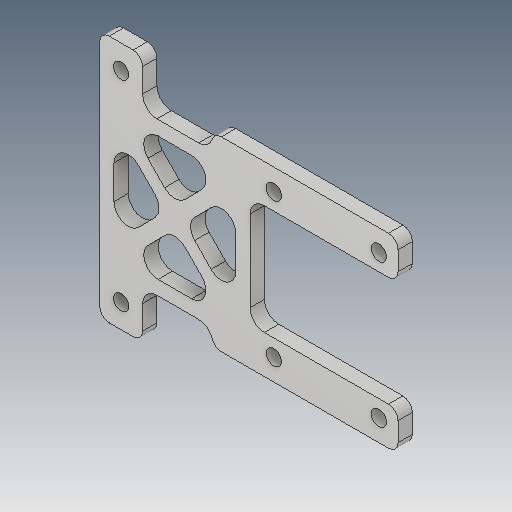
# Autodesk Inventor part: 肩ピッチ固定板_アルミ(A2017)_t3
Saved by Autodesk Inventor 2019.4 (Build 234330000, 330)
## iProperties
Created: 2019-06-27
Part Number: 肩ピッチ固定板_アルミ(A2017)_t3
Material: アルミニウム 2014-T6
Document SubType Name: Modeling
Designer: 長谷川翔一
Density: 2.78927 g/cm^3
Appearance: サテン
Mass: 14.0844 g
Surface Area: 44.3653 cm^2
Volume: 5.04948 cm^3
Author: 長谷川翔一
Autodesk Inventor part; units mm, degrees
ref_plane "YZ Plane" through (0, 0, 0) normal (1, 0, 0) x (0, 1, 0)
ref_plane "XZ Plane" through (0, 0, 0) normal (0, 1, 0) x (-1, 0, 0)
ref_plane "XY Plane" through (0, 0, 0) normal (0, 0, 1) x (1, 0, 0)
sketch "スケッチ1" plane through (0, 0, 0) normal (0, 0, 1) x (1, 0, 0)
  line L0 (7.25, -16) -> (-7.25, -16)
  line L1 (-16.25, -16) -> (-16.25, 16)
  line L2 (-7.25, 16) -> (7.25, 16)
  line L3 (16.25, -16) -> (-16.25, 16) construction
  line L4 (-16.25, -16) -> (16.25, 16) construction
  line L5 (16.25, 0) -> (46.25, 0) construction
  line L6 (46.25, -10.5) -> (16.25, -10.5) construction
  line L7 (16.25, 10.5) -> (46.25, 10.5) construction
  line L8 (46.25, 10.5) -> (46.25, -10.5) construction
  line L9 (46.25, -10.5) -> (16.25, 10.5) construction
  line L10 (16.25, -10.5) -> (46.25, 10.5) construction
  line L11 (46.25, 11.5) -> (15.25, 11.5)
  line L12 (15.25, 11.5) -> (15.25, -11.5)
  line L13 (15.25, -11.5) -> (46.25, -11.5)
  line L14 (46.25, 19.5) -> (7.25, 19.5)
  line L15 (7.25, -19.5) -> (46.25, -19.5)
  line L16 (46.25, 11.5) -> (46.25, 19.5)
  line L17 (46.25, -11.5) -> (46.25, -19.5)
  line L18 (16.25, 10.5) -> (16.25, -10.5) construction
  line L19 (7.25, 19.5) -> (7.25, 16)
  line L20 (7.25, -16) -> (7.25, -19.5)
  line L21 (-16.25, -16) -> (-16.25, -26)
  line L22 (-16.25, -26) -> (-7.25, -26)
  line L23 (-7.25, 26) -> (-16.25, 26)
  line L24 (-16.25, 26) -> (-16.25, 16)
  line L25 (-11.75, 26) -> (-11.75, -26) construction
  line L26 (-11.75, 0) -> (-16.25, 0) construction
  circle A0 centre (-11.75, -21) radius 1.6
  line L27 (-7.25, -26) -> (-7.25, -16)
  line L28 (-7.25, 16) -> (-7.25, 26)
  circle A1 centre (-11.75, 21) radius 1.6
  line L29 (46.25, 10.5) -> (16.25, 10.5) construction
  line L30 (31.25, 10.5) -> (31.25, 19.5) construction
  line L31 (31.25, 15) -> (46.25, 15) construction
  circle A2 centre (37.05, 15) radius 1.6 construction
  circle A3 centre (42.25, 15) radius 1.6
  circle A4 centre (25.45, 15) radius 1.6 construction
  circle A5 centre (20.25, 15) radius 1.6
  circle A6 centre (37.05, -15) radius 1.6 construction
  circle A7 centre (42.25, -15) radius 1.6
  circle A8 centre (25.45, -15) radius 1.6 construction
  circle A9 centre (20.25, -15) radius 1.6
  point P0 (0, 0)
  point P1 (31.25, 0)
  dimension "d21" = 32.5
  dimension "d22" = 32
  dimension "d24" = 30
  dimension "d25" = 21
  dimension "d26" = 1
  dimension "d28" = 30
  dimension "d30" = 9
  dimension "d32" = 9
  dimension "d33" = 3.2
  dimension "d34" = 5
  dimension "d35" = 10
  dimension "d36" = 8
  dimension "d37" = 31
  dimension "d38" = 3.5
  dimension "d39" = 35.5
  dimension "d40" = 9
  dimension "d41" = 3.2
  dimension "d42" = 3.2
  dimension "d43" = 4
  dimension "d44" = 31
  dimension "d46" = 2
  constraints: 64 end point, 11 midpoint, 10 centre point, 9 perpendicular, 7 symmetric about line, 6 parallel, 6 point on line, 3 horizontal, 2 collinear, 2 vertical, 7 other
  measures "d21" distance of L1.end L4.end
  measures "d22" distance of L1.start L1.end
  measures "d24" distance of L7.start L7.end
  measures "d25" distance of L6.end L7.start
  measures "d26" distance between parallel lines of L7 L11
  measures "d28" distance between parallel lines of L8 L18
  measures "d30" distance of L21.end L22.end
  measures "d32" distance of L23.start L23.end
  measures "d33" diameter of A0
  measures "d34" distance from line of L22 A0.centre
  measures "d35" distance between parallel lines of L0 L22
  measures "d36" distance between parallel lines of L15 L13
  measures "d37" distance between parallel lines of L11 L15
  measures "d38" distance between parallel lines of L15 L0
  measures "d39" distance between parallel lines of L15 L2
  measures "d40" distance of L30.start L30.end
  measures "d41" diameter of A2
  measures "d42" diameter of A3
  measures "d43" distance from line of L16 A3.centre
  measures "d44" distance from line of L31.end L12
extrude "押し出し1" add sketch "スケッチ1" along normal blind 3
fillet "フィレット1" radius 2 10 edges at (7.25, 19.5, 1.5) (-7.25, 26, 1.5) (-16.25, 26, 1.5) (46.25, 19.5, 1.5) (46.25, 11.5, 1.5) (46.25, -11.5, 1.5) (46.25, -19.5, 1.5) (7.25, -19.5, 1.5) (-7.25, -26, 1.5) (-16.25, -26, 1.5)
fillet "フィレット2" radius 3 6 edges at (15.25, -11.5, 1.5) (15.25, 11.5, 1.5) (7.25, 16, 1.5) (7.25, -16, 1.5) (-7.25, -16, 1.5) (-7.25, 16, 1.5)
sketch "スケッチ2" plane through (0, 0, 3) normal (0, 0, 1) x (1, 0, 0)
  arc A0 (-16.25, -24) -> (-14.25, -26) centre (-14.25, -24) ccw projected
  line L0 (-14.25, -26) -> (-9.25, -26) projected
  arc A1 (-9.25, -26) -> (-7.25, -24) centre (-9.25, -24) ccw projected
  line L1 (-7.25, -24) -> (-7.25, -19) projected
  arc A2 (-4.25, -16) -> (-7.25, -19) centre (-4.25, -19) ccw projected
  line L2 (-4.25, -16) -> (4.4803, -16) projected
  arc A3 (7.3421, -18.1) -> (4.4803, -16) centre (4.4803, -19) ccw projected
  arc A4 (7.3421, -18.1) -> (9.25, -19.5) centre (9.25, -17.5) ccw projected
  line L3 (9.25, -19.5) -> (44.25, -19.5) projected
  arc A5 (44.25, -19.5) -> (46.25, -17.5) centre (44.25, -17.5) ccw projected
  line L4 (46.25, -17.5) -> (46.25, -13.5) projected
  arc A6 (46.25, -13.5) -> (44.25, -11.5) centre (44.25, -13.5) ccw projected
  line L5 (44.25, -11.5) -> (18.25, -11.5) projected
  arc A7 (15.25, -8.5) -> (18.25, -11.5) centre (18.25, -8.5) ccw projected
  line L6 (15.25, -8.5) -> (15.25, 8.5) projected
  arc A8 (18.25, 11.5) -> (15.25, 8.5) centre (18.25, 8.5) ccw projected
  line L7 (18.25, 11.5) -> (44.25, 11.5) projected
  arc A9 (44.25, 11.5) -> (46.25, 13.5) centre (44.25, 13.5) ccw projected
  line L8 (46.25, 13.5) -> (46.25, 17.5) projected
  arc A10 (46.25, 17.5) -> (44.25, 19.5) centre (44.25, 17.5) ccw projected
  line L9 (44.25, 19.5) -> (9.25, 19.5) projected
  arc A11 (9.25, 19.5) -> (7.3421, 18.1) centre (9.25, 17.5) ccw projected
  arc A12 (4.4803, 16) -> (7.3421, 18.1) centre (4.4803, 19) ccw projected
  line L10 (4.4803, 16) -> (-4.25, 16) projected
  arc A13 (-7.25, 19) -> (-4.25, 16) centre (-4.25, 19) ccw projected
  line L11 (-7.25, 19) -> (-7.25, 24) projected
  arc A14 (-7.25, 24) -> (-9.25, 26) centre (-9.25, 24) ccw projected
  line L12 (-9.25, 26) -> (-14.25, 26) projected
  arc A15 (-14.25, 26) -> (-16.25, 24) centre (-14.25, 24) ccw projected
  line L13 (-16.25, 24) -> (-16.25, -24) projected
  circle A16 centre (42.25, -15) radius 1.6 projected
  circle A17 centre (20.25, -15) radius 1.6 projected
  circle A18 centre (20.25, 15) radius 1.6 projected
  circle A19 centre (42.25, 15) radius 1.6 projected
  circle A20 centre (-11.75, 21) radius 1.6 projected
  circle A21 centre (-11.75, -21) radius 1.6 projected
  circle A22 centre (-11.75, 21) radius 4.6
  circle A23 centre (-11.75, -21) radius 4.6
  line L14 (4.4803, -13) -> (-4.25, -13)
  arc A24 (-9.8384, -16.816) -> (-10.25, -19) centre (-4.25, -19) ccw
  line L15 (-10.25, -19) -> (-10.25, -23)
  line L16 (-10.25, -23) -> (-13.25, -23)
  line L17 (-13.25, 23) -> (-10.25, 23)
  line L18 (-10.25, 23) -> (-10.25, 19)
  arc A25 (-10.25, 19) -> (-9.8384, 16.816) centre (-4.25, 19) ccw
  line L19 (-4.25, 13) -> (4.4803, 13)
  line L20 (9.9347, 16.5) -> (43.25, 16.5)
  line L21 (43.25, 16.5) -> (43.25, 14.5)
  line L22 (43.25, 14.5) -> (18.25, 14.5)
  line L23 (12.25, 8.5) -> (12.25, -8.5)
  arc A26 (14.6318, -13.2863) -> (18.25, -14.5) centre (18.25, -8.5) ccw
  line L24 (18.25, -14.5) -> (43.25, -14.5)
  line L25 (43.25, -14.5) -> (43.25, -16.5)
  line L26 (43.25, -16.5) -> (9.9347, -16.5)
  circle A27 centre (20.25, 15) radius 4.6
  line L27 (-4.25, 13) -> (-11.149, 13)
  line L28 (-4.25, -13) -> (-11.149, -13)
  line L29 (12.25, -8.5) -> (12.25, -10.8578)
  line L30 (12.25, 8.5) -> (12.25, 10.8578)
  line L31 (-13.25, 13) -> (12.25, -13) construction
  line L32 (12.25, 13) -> (-13.25, -13) construction
  line L33 (-13.25, 14.5) -> (-13.25, 23)
  line L34 (4.4803, 13) -> (10.149, 13)
  arc A28 (18.25, 14.5) -> (15.7685, 13.9628) centre (18.25, 8.5) ccw
  line L35 (-13.25, -23) -> (-13.25, -16.6514)
  line L36 (-13.25, -10.8578) -> (-13.25, 10.8578)
  line L37 (10.149, 13) -> (-0.5, 2.1422)
  line L38 (-2.601, 0) -> (-13.25, -10.8578)
  line L39 (-11.149, -13) -> (-0.5, -2.1422)
  line L40 (1.601, 0) -> (12.25, 10.8578)
  line L41 (-13.25, 10.8578) -> (-2.601, 0)
  line L42 (-0.5, -2.1422) -> (10.149, -13)
  line L43 (12.25, -10.8578) -> (1.601, 0)
  line L44 (-0.5, 2.1422) -> (-11.149, 13)
  line L45 (4.4803, -13) -> (10.149, -13)
  arc A29 (9.9347, -16.5) -> (9.3557, -15.5028) centre (4.4803, -19) ccw
  point P0 (0, 0)
  point P1 (-0.5, 0)
  point P2 (-0.5, 0)
  dimension "d51" = 3
  dimension "d52" = 3
  dimension "d53" = 3
  dimension "d54" = 3
  constraints: 68 end point, 13 point on circle, 8 parallel, 6 centre point, 4 perpendicular, 2 midpoint, 2 point on line, 1 horizontal, 1 tangent, 12 other
  measures "d52" radial gap between concentric circles of A21 A23
  measures "d53" distance between parallel lines of L2 L14
extrude "押し出し2" cut sketch "スケッチ2" against normal through all contours L14 L28 L39 L42 L45 | L19 L34 L37 L44 L27 | L23 L29 L43 L40 L30 | L36 L41 L38
fillet "フィレット3" radius 3 12 edges at (-11.149, 13, 1.5) (10.149, 13, 1.5) (-0.5, 2.1422, 1.5) (-13.25, 10.8578, 1.5) (-13.25, -10.8578, 1.5) (-2.601, 0, 1.5) (-0.5, -2.1422, 1.5) (-11.149, -13, 1.5) (10.149, -13, 1.5) (1.601, 0, 1.5) (12.25, 10.8578, 1.5) (12.25, -10.8578, 1.5)
